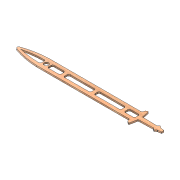
# Autodesk Inventor part: Romeo And Juliette Sword_LONG
Saved by Autodesk Inventor 2021 (Build 250183000, 183)
## iProperties
Created: 2018-05-23
Part Number: Romeo And Juliette Sword_LONG
Material: Wood (Birch)
Document SubType Name: Modeling
Designer: dbrui
Density: 0.55 g/cm^3
Appearance: Birch - Natural Polished
Author: dbrui
Autodesk Inventor part; units mm, degrees
ref_plane "YZ Plane" through (0, 0, 0) normal (1, 0, 0) x (0, 1, 0)
ref_plane "XZ Plane" through (0, 0, 0) normal (0, 1, 0) x (-1, 0, 0)
ref_plane "XY Plane" through (0, 0, 0) normal (0, 0, 1) x (1, 0, 0)
sketch "Sketch1" plane through (0, 0, 0) normal (0, 1, 0) x (-1, 0, 0)
  line L0 (457.2, 76.2) -> (-457.2, 76.2) construction
  line L1 (-457.2, 76.2) -> (-457.2, -76.2) construction
  line L2 (-457.2, -76.2) -> (457.2, -76.2) construction
  line L3 (457.2, -76.2) -> (457.2, 76.2) construction
  line L4 (457.2, 76.2) -> (-457.2, -76.2) construction
  line L5 (-457.2, 76.2) -> (457.2, -76.2) construction
  line L6 (-457.2, 7.9375) -> (-457.2, -7.9375)
  line L7 (-457.2, -7.9375) -> (-432.0472, -11.4725)
  line L8 (-457.2, -7.9375) -> (-431.8, -7.9375) construction
  line L9 (-457.2, 7.9375) -> (-432.0472, 11.4725)
  line L10 (-457.2, 7.9375) -> (-431.8, 7.9375) construction
  line L11 (-432.0472, 11.4725) -> (-432.0472, -11.4725)
  line L12 (-432.0472, 11.4725) -> (-419.3472, 21.8097)
  line L13 (-419.3472, 21.8097) -> (-419.3472, -21.8097)
  line L14 (-419.3472, -21.8097) -> (-432.0472, -11.4725)
  line L15 (-406.6472, 11.4725) -> (-406.6472, -11.4725)
  line L16 (-406.6472, 11.4725) -> (-419.3472, 21.8097)
  line L17 (-419.3472, -21.8097) -> (-406.6472, -11.4725)
  line L18 (-324.0972, 13.5255) -> (-324.0972, -13.5255)
  line L19 (-324.0972, 13.5255) -> (-406.6472, 11.4725)
  line L20 (-324.0972, -13.5255) -> (-406.6472, -11.4725)
  line L21 (-324.0972, 13.5255) -> (-298.6972, 13.5255) construction
  line L22 (-324.0972, -13.5255) -> (-298.6972, -13.5255) construction
  line L23 (-406.6472, 0) -> (-401.5952, 0)
  line L24 (44.2028, 13.5255) -> (44.2028, -13.5255)
  line L25 (-244.337, 13.5255) -> (44.2028, 13.5255)
  line L26 (44.2028, -13.5255) -> (-244.337, -13.5255)
  arc A0 (120.4028, 0) -> (44.2028, 13.5255) centre (44.2028, -207.8851) ccw
  arc A1 (44.2028, -13.5255) -> (120.4028, 0) centre (44.2028, 207.8851) ccw
  arc A2 (-244.337, -13.5255) -> (-254.0713, -10.3505) centre (-254.0713, -26.8605) ccw
  arc A3 (-254.0713, 10.3505) -> (-244.337, 13.5255) centre (-254.0713, 26.8605) ccw
  line L27 (-254.0713, -10.3505) -> (-269.9463, -10.3505)
  line L28 (-254.0713, 10.3505) -> (-269.9463, 10.3505)
  line L29 (-298.6947, -64.7889) -> (-285.8213, -64.7889)
  line L30 (-285.8213, -64.7889) -> (-269.9463, -10.3505)
  line L31 (-298.6947, 64.7889) -> (-285.8213, 64.7889)
  line L32 (-285.8213, 64.7889) -> (-269.9463, 10.3505)
  line L33 (-324.0972, -13.5255) -> (-318.7941, -13.5255)
  line L34 (-324.0972, 13.5255) -> (-318.7941, 13.5255)
  line L35 (-308.7454, -13.5255) -> (-298.6947, -64.7889)
  line L36 (-308.7454, 13.5255) -> (-298.6947, 64.7889)
  line L37 (-324.0972, -13.5255) -> (-308.7454, -13.5255)
  line L38 (-324.0972, 13.5255) -> (-308.7454, 13.5255)
  point P0 (0, 0)
  point P1 (-457.2, 0)
  point P2 (-457.2, 0)
  point P3 (44.2028, 0)
  point P4 (0, 0)
  point P5 (0, 0)
  dimension "d0" = 914.4
  dimension "d1" = 152.4
  dimension "d3" = 15.875
  dimension "d4" = 25.4
  dimension "d5" = 8
  dimension "d6" = 25.4
  dimension "d7" = 8
  dimension "d8" = 12.7
  dimension "d9" = 16.3752
  dimension "d10" = 16.3752
  dimension "d11" = 27.051
  dimension "d25" = 27.051
  dimension "d27" = 76.2
  dimension "d37" = 16.51
  dimension "d38" = 16.51
  dimension "d63" = 3.175
  dimension "d64" = 3.175
  dimension "d71" = 56.7059
  dimension "d72" = 56.7059
  dimension "d73" = 12.8734
  dimension "d74" = 12.8734
  dimension "d75" = 52.2394
  dimension "d76" = 52.2394
  dimension "d77" = 27.35
  dimension "d78" = 412.9972
  dimension "d79" = 256.2545
  dimension "d80" = 701.537
  dimension "d81" = 701.537
  dimension "d82" = 755.8972
  dimension "d83" = 755.8972
  dimension "d84" = 775.9941
  dimension "d85" = 775.9941
  dimension "d86" = 858.7952
  dimension "d87" = 16.257
  dimension "d88" = 88.575
  constraints: 78 end point, 10 horizontal, 8 midpoint, 8 point on circle, 6 horizontal alignment, 6 point on line, 4 centre point, 4 tangent, 4 vertical, 3 parallel, 3 symmetric about line, 2 coincident, 2 equal length, 1 perpendicular
  measures "d0" distance of L2.end L1.end
  measures "d1" distance of L1.end L0.end
  measures "d3" distance of L6.start L6.end
  measures "d4" distance of L6.end L7.end
  measures "d5" angle of L7 L8
  measures "d6" distance of L6.start L9.end
  measures "d7" angle of L10 L9
  measures "d8" horizontal distance of L9.end L12.end
  measures "d9" distance of L9.end L12.end
  measures "d10" distance of L13.end L7.end
  measures "d11" distance of L18.start L18.end
  measures "d25" distance of L24.start L24.end
  measures "d27" distance of point (44.203, 0) A0.start
  measures "d37" radius of A3
  measures "d38" radius of A2
  measures "d63" distance between parallel lines of L25 L28
  measures "d64" distance between parallel lines of L26 L27
  measures "d71" distance of L31.end L28.end
  measures "d72" distance of L29.end L27.end
  measures "d73" distance of L29.start L29.end
  measures "d74" distance of L31.start L31.end
  measures "d75" distance of L36.start L31.start
  measures "d76" distance of L35.start L29.start
  measures "d77" angle of L35 L30
  measures "d78" distance between parallel lines of L3 L24
  measures "d79" distance from line of point (0, 0) L32
  measures "d80" distance from line of L25.start L3
  measures "d81" distance from line of L26.end L3
  measures "d82" distance from line of L21.end L3
  measures "d83" distance from line of L22.end L3
  measures "d84" distance from line of L34.end L3
  measures "d85" distance from line of L33.end L3
  measures "d86" distance from line of L23.end L3
  measures "d87" angle of L32 L3
  measures "d88" angle of L19 L3
extrude "Extrusion4" add sketch "Sketch1" along normal blind 3.175
chamfer "Chamfer2" distance 3.175 angle 45 3 edges at (298.6947, 1.5875, 64.7889) (298.6947, 1.5875, -64.7889) (308.7454, 1.5875, 13.5255)
fillet "Fillet4" radius 1.651 11 edges at (254.0713, 1.5875, 10.3505) (254.0713, 1.5875, -10.3505) (-120.4028, 1.5875, 0) (457.2, 1.5875, 7.9375) (432.0472, 1.5875, 11.4725) (419.3472, 1.5875, 21.8097) (406.6472, 1.5875, 11.4725) (457.2, 1.5875, -7.9375) (419.3472, 1.5875, -21.8097) (432.0472, 1.5875, -11.4725) (406.6472, 1.5875, -11.4725)
fillet "Fillet6" radius 6.35 2 edges at (324.0972, 1.5875, 13.5255) (324.0972, 1.5875, -13.5255)
chamfer "Chamfer3" distance 7.9375 angle 45 4 edges at (269.9463, 1.5875, 10.3505) (285.8213, 1.5875, 64.7889) (285.8213, 1.5875, -64.7889) (269.9463, 1.5875, -10.3505)
sketch "Sketch2" plane through (0, 3.175, 0) normal (0, 1, 0) x (1, 0, 0)
  line L0 (278.5925, 40) -> (-521.4075, 40)
  line L1 (-521.4075, 40) -> (-521.4075, -40)
  line L2 (-521.4075, -40) -> (278.5925, -40)
  line L3 (278.5925, -40) -> (278.5925, 40)
  line L4 (283.5992, 57.1688) -> (272.1685, 17.9706) projected
  arc A0 (-521.4075, 0) -> (-294.5562, -40) centre (-314.028, 512.8385) ccw
  line L5 (-521.4075, 0) -> (-294.5562, -40) construction
  line L6 (-521.4075, 0) -> (-291.0566, 0) construction
  arc A1 (-294.5562, 40) -> (-521.4075, 0) centre (-314.0281, -512.8382) ccw
  line L7 (-294.5562, 40) -> (-294.5562, -40)
  point P0 (0, 0)
  point P1 (-333.5, 40)
  point P2 (-333.4998, -40)
  dimension "d89" = 800
  dimension "d90" = 80
  dimension "d91" = 40
  dimension "d92" = 10
  dimension "d93" = 553.181
  constraints: 14 end point, 4 point on circle, 3 point on line, 2 centre point, 2 horizontal, 2 parallel, 2 perpendicular, 1 equal length, 1 midpoint
  measures "d89" distance of L2.end L1.end
  measures "d90" distance of L1.end L0.end
  measures "d91" distance from line of point (0, 0) L0
  measures "d92" angle of L5 L6
  measures "d93" radius of A1
extrude "Extrusion5" add sketch "Sketch2" against normal up to surface (3.175 mm away) contours L3 L2 L7 L0 | L7 L2 A0 A1 L0
fillet "Fillet8" radius 10 1 edges at (-521.4075, 1.5875, 0)
fillet "Fillet9" radius 10 2 edges at (278.5925, 1.5875, 40) (278.5925, 1.5875, -40)
sketch "Sketch3" plane through (0, 3.175, 0) normal (0, 1, 0) x (1, 0, 0)
  arc A0 (-496.328, 9.4414) -> (-496.328, -9.4414) centre (-493.0325, 0) ccw projected
  arc A1 (-496.328, -9.4414) -> (-333.4998, -40) centre (-314.028, 512.8385) ccw projected
  line L0 (-333.4998, -40) -> (271.0922, -40) projected
  arc A2 (280.6923, -47.2005) -> (271.0922, -40) centre (271.0922, -50) ccw projected
  line L1 (280.6923, -47.2005) -> (283.5992, -57.1688) projected
  line L2 (293.7588, -64.7889) -> (283.5992, -57.1688) projected
  line L3 (293.7588, -64.7889) -> (295.5197, -64.7889) projected
  line L4 (299.3055, -61.6732) -> (295.5197, -64.7889) projected
  line L5 (299.3055, -61.6732) -> (308.1345, -16.6412) projected
  line L6 (311.9204, -13.5255) -> (308.1345, -16.6412) projected
  line L7 (311.9204, -13.5255) -> (324.0182, -13.5255) projected
  arc A3 (324.0182, -13.5255) -> (324.1761, -13.5235) centre (324.0182, -7.1755) ccw projected
  line L8 (324.1761, -13.5235) -> (406.0372, -11.4877) projected
  arc A4 (407.1204, -11.8577) -> (406.0372, -11.4877) centre (406.0782, -13.1382) ccw projected
  line L9 (407.1204, -11.8577) -> (418.305, -20.9614) projected
  arc A5 (418.305, -20.9614) -> (420.3894, -20.9614) centre (419.3472, -19.6809) ccw projected
  line L10 (420.3894, -20.9614) -> (431.6904, -11.7629) projected
  arc A6 (432.5028, -11.4085) -> (431.6904, -11.7629) centre (432.7326, -13.0434) ccw projected
  line L11 (432.5028, -11.4085) -> (455.7788, -8.1372) projected
  arc A7 (455.7788, -8.1372) -> (457.2, -6.5023) centre (455.549, -6.5023) ccw projected
  line L12 (457.2, -6.5023) -> (457.2, 6.5023) projected
  arc A8 (457.2, 6.5023) -> (455.7788, 8.1372) centre (455.549, 6.5023) ccw projected
  line L13 (455.7788, 8.1372) -> (432.5028, 11.4085) projected
  arc A9 (431.6904, 11.7629) -> (432.5028, 11.4085) centre (432.7326, 13.0434) ccw projected
  line L14 (431.6904, 11.7629) -> (420.3894, 20.9614) projected
  arc A10 (420.3894, 20.9614) -> (418.305, 20.9614) centre (419.3472, 19.6809) ccw projected
  line L15 (418.305, 20.9614) -> (407.1204, 11.8577) projected
  arc A11 (406.0372, 11.4877) -> (407.1204, 11.8577) centre (406.0782, 13.1382) ccw projected
  line L16 (406.0372, 11.4877) -> (324.1761, 13.5235) projected
  arc A12 (324.1761, 13.5235) -> (324.0182, 13.5255) centre (324.0182, 7.1755) ccw projected
  line L17 (324.0182, 13.5255) -> (308.7454, 13.5255) projected
  line L18 (308.7454, 13.5255) -> (299.3055, 61.6732) projected
  line L19 (295.5197, 64.7889) -> (299.3055, 61.6732) projected
  line L20 (295.5197, 64.7889) -> (293.7588, 64.7889) projected
  line L21 (283.5992, 57.1688) -> (293.7588, 64.7889) projected
  line L22 (283.5992, 57.1688) -> (280.6923, 47.2005) projected
  arc A13 (271.0922, 40) -> (280.6923, 47.2005) centre (271.0922, 50) ccw projected
  line L23 (271.0922, 40) -> (-333.5, 40) projected
  arc A14 (-333.5, 40) -> (-496.328, 9.4414) centre (-314.0281, -512.8382) ccw projected
  point P0 (0, 0)
extrude "Extrusion6" add sketch "Sketch3" along normal blind 6.825
sketch "Sketch4" plane through (0, 10, 0) normal (0, 1, 0) x (1, 0, 0)
  line L0 (287.5, 17.5725) -> (-287.5, 17.5725)
  line L1 (-287.5, 17.5725) -> (-287.5, -17.5725)
  line L2 (-287.5, -17.5725) -> (287.5, -17.5725)
  line L3 (287.5, -17.5725) -> (287.5, 17.5725)
  line L4 (287.5, 17.5725) -> (-287.5, -17.5725) construction
  line L5 (-287.5, 17.5725) -> (287.5, -17.5725) construction
  line L6 (-287.5, 17.5725) -> (-333.4998, 17.5725)
  line L7 (-333.4998, 17.5725) -> (-333.4998, -17.5725)
  line L8 (-333.4998, -17.5725) -> (-287.5, -17.5725)
  line L9 (-287.5, -17.5725) -> (-287.5, 17.5725)
  arc A0 (-333.4998, 17.5725) -> (-480.605, 0) centre (-340.8548, -545.3758) ccw
  arc A1 (-480.605, 0) -> (-333.4998, -17.5725) centre (-337.1773, 576.1611) ccw
  point P0 (0, 0)
  dimension "d100" = 575
  constraints: 20 end point, 4 parallel, 4 point on circle, 2 centre point, 2 horizontal, 2 midpoint, 2 perpendicular
  measures "d100" distance of L2.end L1.end
extrude "Extrusion7" cut sketch "Sketch4" against normal blind 10 contours L3 L2 L1 L0 | L7 A1 A0
fillet "Fillet10" radius 10 6 edges at (-333.4998, 5, -17.5725) (-333.4998, 5, 17.5725) (-287.5, 5, -17.5725) (-287.5, 5, 17.5725) (287.5, 5, 17.5725) (287.5, 5, -17.5725)
sketch "Sketch5" plane through (0, 10, 0) normal (0, 1, 0) x (1, 0, 0)
  circle A0 centre (-310.5, 0.0323) radius 15
  line L0 (-287.5, -7.5725) -> (-287.5, 7.5725) projected
  point P0 (0, 0)
  dimension "d104" = 30
  dimension "d105" = 23
  constraints: 1 centre point
  measures "d104" diameter of A0
  measures "d105" distance from line of L0 A0.centre
extrude "Extrusion8" cut sketch "Sketch5" against normal through all
sketch "Sketch6" plane through (0, 10, 0) normal (0, 1, 0) x (1, 0, 0)
  line L0 (-277.5, -17.5725) -> (277.5, -17.5725) projected
  line L1 (218.714, 17.5725) -> (196.286, 17.5725)
  line L2 (196.286, 17.5725) -> (196.286, -17.5725)
  line L3 (196.286, -17.5725) -> (218.714, -17.5725)
  line L4 (218.714, -17.5725) -> (218.714, 17.5725)
  line L5 (218.714, 17.5725) -> (196.286, -17.5725) construction
  line L6 (196.286, 17.5725) -> (218.714, -17.5725) construction
  line L7 (287.5, 7.5725) -> (287.5, -7.5725) projected
  point P0 (0, 0)
  point P1 (207.5, 0)
  dimension "d108" = 22.428
  dimension "d109" = 80
  constraints: 12 end point, 2 midpoint, 2 parallel, 1 horizontal, 1 perpendicular, 1 point on line
  measures "d108" distance of L3.end L2.end
  measures "d109" distance from line of L7 point (207.5, 0)
extrude "Extrusion9" add sketch "Sketch6" against normal blind 10
fillet "Fillet11" radius 10 4 edges at (196.286, 5, -17.5725) (196.286, 5, 17.5725) (218.714, 5, 17.5725) (218.714, 5, -17.5725)
pattern_linear "Rectangular Pattern1" count 3 spacing 200 along (-1, 0, 0) of "Extrusion9", "Fillet11"
equation "\"d4\" = d6"
equation "\"d7\" = d5"
equation "\"d10\" = d9"
equation "\"d25\" = d11"
equation "\"d38\" = d37"
equation "\"d64\" = d63"
body "Solid3"
